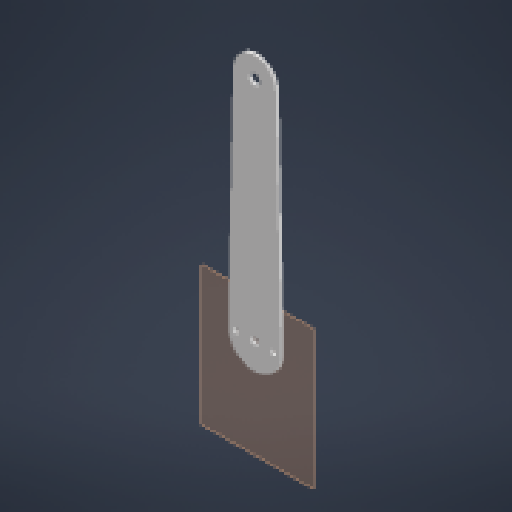
# Autodesk Inventor part: Link2Base2
Saved by Autodesk Inventor 2023 (Build 270158000, 158)
## iProperties
Created: 2023-09-09
Part Number: Link2Base2
Material: Generic
Document SubType Name: Modeling
Designer: philo
Density: 1 g/cm^3
Appearance: Default
Mass: 33.5041 g
Surface Area: 242.108 cm^2
Volume: 33.5041 cm^3
Author: philo
Autodesk Inventor part; units mm, degrees
ref_plane "YZ Plane" through (0, 0, 0) normal (1, 0, 0) x (0, 1, 0)
ref_plane "XZ Plane" through (0, 0, 0) normal (0, 1, 0) x (-1, 0, 0)
ref_plane "XY Plane" through (0, 0, 0) normal (0, 0, 1) x (1, 0, 0)
ref_plane "Work Plane2" through (0.4904, 0, 14) normal (0, 0, 1) x (1, 0, 0)
sketch "Sketch1" plane through (0.4904, 0, 14) normal (0, 0, 1) x (1, 0, 0)
  line L0 (-25, 245.7065) -> (25, 245.7065)
  line L1 (25, 245.7065) -> (25, 5.7065)
  line L2 (25, 5.7065) -> (-25, 5.7065)
  line L3 (-25, 5.7065) -> (-25, 245.7065)
  line L4 (-20, 245.7065) -> (20, 245.7065)
  line L5 (20, 5.7065) -> (-20, 5.7065)
  circle A0 centre (0, 30.7065) radius 3.5 projected
  circle A1 centre (0, 30.7065) radius 25
  circle A2 centre (0, 245.7065) radius 20
  line L6 (-25, 30.7065) -> (-20, 245.7065)
  line L7 (20, 245.7065) -> (25, 30.7065)
  point P0 (-0.4904, 0)
  point P1 (-20, 245.7065)
  dimension "d6" = 240
  dimension "d7" = 0
  dimension "d9" = 50
  dimension "d10" = 25
  dimension "d11" = 25
  dimension "d12" = 25
  dimension "d13" = 0
  constraints: 16 end point, 3 parallel, 2 horizontal, 2 point on circle, 2 point on line, 1 centre point, 1 coincident, 1 midpoint, 1 perpendicular, 3 other
  measures "d6" distance between parallel lines of L2 L0
  measures "d7" distance between parallel lines of L0 L4
  measures "d9" diameter of A1
  measures "d10" distance from line of L3 A1.centre
  measures "d11" distance from line of L1 A1.centre
  measures "d12" distance from line of A1.centre L2
  measures "d13" distance between parallel lines of L5 L2
extrude "Extrusion1" add sketch "Sketch1" along normal blind 3 contours A2 L0 | L0 A2 | A2 L7 A1 L6 | L6 A1 L7
sketch "Sketch2" plane through (0.4904, 0, 17) normal (0, 0, 1) x (1, 0, 0)
  arc A0 (20, 245.7065) -> (-20, 245.7065) centre (0, 245.7065) ccw projected
  circle A1 centre (0, 245.7065) radius 5
  point P0 (-0.4904, 0)
  dimension "d16" = 10
  constraints: 1 centre point, 1 coincident
  measures "d16" diameter of A1
extrude "Extrusion2" cut sketch "Sketch2" against normal blind 3
sketch "Sketch3" plane through (0.4904, 0, 17) normal (0, 0, 1) x (1, 0, 0)
  circle A0 centre (-9.4508, 46.0264) radius 2.5 projected
  circle A1 centre (8.7917, 14.9991) radius 2.5 projected
  point P0 (-0.4904, 0)
extrude "Extrusion3" cut sketch "Sketch3" against normal blind 10
body "Solid1"
